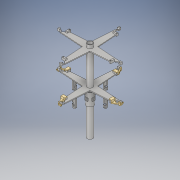
# Autodesk Inventor part: Center beam
Saved by Autodesk Inventor 2018.1 (Build 221171000, 171)
## iProperties
Created: 2017-09-02
Part Number: Center beam
Material: Generic
Document SubType Name: Modeling
Designer: ToreDenStore
Density: 1 g/cm^3
Appearance: Default
Author: ToreDenStore
Autodesk Inventor part; units mm, degrees
sketch "Sketch1" plane through (0, 0, 0) normal (0, 1, 0) x (-1, 0, 0)
  circle A0 centre (0, 0) radius 10
  circle A1 centre (0, 0) radius 8
  dimension "d0" = 20
  dimension "d1" = 2
  constraints: 2 centre point, 2 coincident
  measures "d0" diameter of A0
  measures "d1" radial gap between concentric circles of A0 A1
extrude "Extrusion1" add sketch "Sketch1" along normal blind 300
ref_plane "Work Plane1" through (0, 105, 0) normal (0, -1, 0) x (1, 0, 0)
sketch "Sketch2" plane through (0, 105, 0) normal (0, -1, 0) x (1, 0, 0)
  circle A0 centre (0, 0) radius 12.5
  circle A1 centre (0, 0) radius 10 projected
  dimension "d5" = 25
  constraints: 1 centre point, 1 coincident
  measures "d5" diameter of A0
extrude "Extrusion2" add sketch "Sketch2" against normal blind 45
ref_plane "Work Plane8" through (0, 127.5, 0) normal (0, 1, 0) x (1, 0, 0)
sketch "Sketch19" plane through (0, 127.5, 0) normal (0, 1, 0) x (1, 0, 0)
  circle A0 centre (0, 0) radius 12.5
  line L0 (-5, 11.456439) -> (-5, 14.456439)
  line L1 (-5, 14.456439) -> (5, 14.456439)
  line L2 (5, 14.456439) -> (5, 11.456439)
  line L3 (0, 19.847727) -> (0, -17.891288)
  dimension "d107" = 10
  dimension "d108" = 3
  dimension "d109" = 5
  constraints: 6 end point, 2 perpendicular, 2 point on circle, 1 vertical
  measures "d107" distance of L0.end L1.end
  measures "d108" distance of L1.end L2.end
  measures "d109" distance between parallel lines of L2 L3
extrude "Extrusion12" add sketch "Sketch19" along normal mid plane 10 contours A0 L3 L1 L2 | A0 L0 L1 L3
sketch "Sketch20" plane through (5, 132.5, -14.456439) normal (0, 0, -1) x (-1, 0, 0)
  line L0 (0, 0) -> (10, 0) projected
  line L1 (10, -10) -> (10, 0) projected
  point P0 (5, -132.5)
  point P1 (5, -6)
  dimension "d112" = 6
  dimension "d113" = 5
  measures "d112" distance from line of L0 point (5, -6)
  measures "d113" distance from line of point (5, -6) L1
hole "Hole4" at (0, 126.5, -14.456439) direction (0, 0, 1) diameter 5 depth 8 tip angle 118
pattern_circular "Circular Pattern6" count 4 over 360 about axis through (0, 0, 0) along (0, 1, 0) of "Hole4", "Extrusion12"
ref_plane "Work Plane9" through (0, 160, 0) normal (0, 1, 0) x (1, 0, 0)
sketch "Sketch3" plane through (0, 160, 0) normal (0, 1, 0) x (1, 0, 0)
  circle A0 centre (0, 0) radius 10
  line L0 (0, 0) -> (-10, 0) construction
  line L1 (-15, 0) -> (-7.98058, 100.557087)
  line L2 (7.98058, 100.557087) -> (15, 0)
  line L3 (15, 0) -> (10, 0)
  line L4 (0, 0) -> (0, 100) construction
  arc A1 (7.98058, 100.557087) -> (-7.98058, 100.557087) centre (0, 100) ccw
  circle A2 centre (0, 100) radius 5
  line L5 (10, 0) -> (0, 0) construction
  line L6 (-10, 0) -> (-15, 0)
  dimension "d9" = 15
  dimension "d10" = 100
  dimension "d11" = 8
  dimension "d12" = 10
  constraints: 14 end point, 4 collinear, 4 point on circle, 2 centre point, 2 coincident, 2 horizontal, 2 tangent, 1 equal length, 1 point on line, 1 vertical
  measures "d9" distance of L2.end L0.start
  measures "d10" distance of L0.start L4.end
  measures "d11" radius of A1
  measures "d12" diameter of A2
extrude "Extrusion3" add sketch "Sketch3" along normal blind 3 contours A0 L6 L1 A1 L2 L3
pattern_circular "Circular Pattern1" count 4 over 360 about axis through (0, 0, 0) along (0, 1, 0) of "Extrusion3"
sketch "Sketch9" plane through (0, 163, 0) normal (0, 1, 0) x (1, 0, 0)
  circle A0 centre (0, 100) radius 5
  arc A1 (7.98058, 100.557087) -> (-7.98058, 100.557087) centre (0, 100) ccw
  line L0 (0, 108) -> (0, 105)
  line L1 (0, 95) -> (0, 90)
  line L2 (0, 90) -> (8.717521, 90)
  line L3 (14.021243, 14.021243) -> (7.98058, 100.557087)
  point P0 (0, 0)
  dimension "d59" = 5
  constraints: 6 end point, 3 point on circle, 3 point on line, 1 perpendicular
  measures "d59" distance of L1.start L1.end
extrude "Extrusion7" cut sketch "Sketch9" against normal blind 5 contours A0 L0 A1 L3 L2 L1
sketch "Sketch11" plane through (0, 163, 0) normal (0, 1, 0) x (1, 0, 0)
  line L0 (0, 90) -> (8.717521, 90)
  line L1 (8.717521, 90) -> (13.717521, 90)
  line L2 (13.717521, 90) -> (13.717521, 84)
  line L3 (13.717521, 84) -> (9.136353, 84)
  arc A0 (0, 108) -> (-7.98058, 100.557087) centre (0, 100) ccw
  line L4 (0, 108) -> (0, 113)
  line L5 (0, 113) -> (-6, 113)
  line L6 (-6, 113) -> (-6, 105.291503)
  line L7 (14.021243, 14.021243) -> (8.717521, 90)
  point P0 (0, 0)
  dimension "d62" = 5
  dimension "d63" = 6
  dimension "d64" = 5
  dimension "d65" = 6
  constraints: 12 end point, 4 perpendicular, 1 horizontal, 1 point on circle, 1 point on line, 1 vertical
  measures "d62" distance of L0.end L1.end
  measures "d63" distance of L1.end L2.end
  measures "d64" distance of L4.start L4.end
  measures "d65" distance of L4.end L5.end
extrude "Extrusion8" add sketch "Sketch11" against normal blind 3
sketch "Sketch13" plane through (0, 163, 0) normal (0, 1, 0) x (1, 0, 0)
  line L0 (0, 113) -> (0, 105)
  line L1 (-6, 113) -> (0, 113)
  arc A0 (-6, 105.291503) -> (-7.98058, 100.557087) centre (0, 100) ccw
  line L2 (13.717521, 90) -> (0, 90)
  line L3 (13.717521, 90) -> (13.717521, 84)
  line L4 (13.717521, 84) -> (9.136353, 84)
  line L5 (14.021243, 14.021243) -> (9.136353, 84)
  circle A1 centre (0, 100) radius 5
  line L6 (-6, 105.291503) -> (-6, 113)
  arc A2 (-6, 105.291503) -> (-7.98058, 100.557087) centre (0, 100) ccw
  line L7 (-3, 105.291503) -> (-3, 104)
  arc A3 (0, 105) -> (0, 95) centre (0, 100) ccw
  line L8 (9.136353, 84) -> (0, 84)
  line L9 (0, 84) -> (0, 90)
  point P0 (0, 0)
  point P1 (7.98058, 100.557087)
  constraints: 6 end point, 2 vertical, 1 horizontal, 1 point on circle
sketch "Sketch13 outline for Extrusion9" plane through (0, 163, 0) normal (0, 1, 0) x (1, 0, 0)
  line L0 (0, 105) -> (0, 113)
  arc A0 (-3, 104) -> (0, 105) centre (0, 100) cw
  line L1 (-6, 105.291503) -> (-3, 104)
  line L2 (-6, 113) -> (-6, 105.291503)
  line L3 (0, 113) -> (-6, 113)
  line L4 (0, 84) -> (13.717521, 84)
  line L5 (13.717521, 84) -> (13.717521, 90)
  line L6 (13.717521, 90) -> (0, 90)
  line L7 (0, 90) -> (0, 84)
extrude "Extrusion9" add sketch "Sketch13 outline for Extrusion9" along normal blind 5
sketch "Sketch21" plane through (0, 168, 0) normal (0, 1, 0) x (1, 0, 0)
  line L0 (13.717521, 84) -> (13.717521, 90)
  line L1 (13.717521, 90) -> (0, 90)
  point P0 (0, 0)
  point P1 (10.717521, 87)
  dimension "d141" = 3
  dimension "d142" = 3
  measures "d141" distance from line of L1 point (10.718, 87)
  measures "d142" distance from line of L0 point (10.718, 87)
hole "Hole5" at (10.717521, 168, -87) direction (0, -1, 0) diameter 3 depth 4
sketch "Sketch22" plane through (10.717521, 164, -87) normal (0, 1, 0) x (1, 0, 0)
  circle A0 centre (0, 0) radius 1.5 projected
  point P0 (-10.717521, -87)
extrude "Extrusion15" add sketch "Sketch22" along normal blind 4 separate body
sketch "Sketch23" plane through (10.717521, 168, -87) normal (0, 1, 0) x (1, 0, 0)
  line L0 (3, 3) -> (-10.717521, 3)
  line L1 (3, -3) -> (3, 3)
  line L2 (-10.717521, -3) -> (3, -3)
  line L3 (-10.717521, 3) -> (-10.717521, -3)
  point P0 (-10.717521, -87)
extrude "Extrusion16" add sketch "Sketch23" along normal blind 3 bodies 2
sketch "Sketch18" plane through (0, 163, 0) normal (0, 1, 0) x (1, 0, 0)
  arc A0 (-3, 104) -> (0, 95) centre (0, 100) ccw projected
  circle A1 centre (0, 100) radius 8
  point P0 (0, 0)
  dimension "d97" = 16
  constraints: 1 centre point, 1 coincident
  measures "d97" diameter of A1
extrude "Extrusion11" cut sketch "Sketch18" along normal blind 5 bodies 1
sketch "Sketch24" plane through (13.717521, 168, -90) normal (0, 0, -1) x (-1, 0, 0)
  line L0 (13.717521, 3) -> (0, 3)
  line L1 (0, 0) -> (0, -8)
  line L2 (0, 0) -> (0, 3)
  line L3 (13.717521, 0) -> (13.717521, 3)
  line L4 (13.717521, -5) -> (13.717521, 0)
  line L5 (3.717521, -8) -> (23.717521, -8)
  line L6 (0, -8) -> (4.581168, -8)
  line L7 (13.717521, -5) -> (13.717521, -8)
  point P0 (13.717521, -168)
  constraints: 2 end point, 1 midpoint
extrude "Extrusion17" add sketch "Sketch24" along normal blind 3 bodies 2
sketch "Sketch25" plane through (0, 160, -90) normal (0, -1, 0) x (1, 0, 0)
  arc A0 (0, -5) -> (0, -15) centre (0, -10) ccw
  line L0 (0, -23) -> (0, -15)
  line L1 (0, -5) -> (0, 0)
  line L2 (13.717521, -3) -> (0, -3)
  circle A1 centre (0, -10) radius 5
  line L3 (0, -23) -> (3, -23)
  circle A2 centre (0, -10) radius 8
  line L4 (13.717521, -3) -> (6.808814, -14.200006)
  line L5 (3, -23) -> (3, -17.416198)
  point P0 (0, 90)
  dimension "d172" = 10
  dimension "d173" = 3
  dimension "d174" = 16
  constraints: 6 end point, 2 centre point, 2 coincident, 2 point on circle, 1 horizontal, 1 tangent, 1 vertical
  measures "d172" diameter of A1
  measures "d173" distance of L0.start L3.end
  measures "d174" diameter of A2
extrude "Extrusion22" add sketch "Sketch25" against normal blind 3 contours L1 L2 A2 L0 A1 | A2 L5 L3 L0 | L2 L4 A2 bodies 2
sketch "Sketch30" plane through (0, 160, -90) normal (0, -1, 0) x (1, 0, 0)
  line L0 (3, -23) -> (3, -17.416198)
  line L1 (0, -23) -> (3, -23)
  line L2 (-6, -23) -> (0, -23)
  line L3 (-6, -15.291503) -> (-6, -23)
  line L4 (3, -19) -> (-6, -19)
  point P0 (0, 90)
  dimension "d177" = 4
  constraints: 2 end point, 2 point on line, 1 perpendicular
  measures "d177" distance between parallel lines of L1 L4
extrude "Extrusion23" add sketch "Sketch30" along normal blind 3 bodies 2
sketch "Sketch31" plane through (0, 163, -90) normal (0, 1, 0) x (1, 0, 0)
  line L0 (0, 18) -> (0, 23)
  line L1 (3, 23) -> (0, 23)
  line L2 (3, 17.416198) -> (3, 23)
  line L3 (0, 18) -> (0, 15)
  line L4 (0, 18) -> (3, 17.416198)
  point P0 (0, -90)
  constraints: 2 end point
extrude "Extrusion24" add sketch "Sketch31" along normal blind 5 bodies 2
sketch "Sketch32" plane through (0, 163, -90) normal (0, 1, 0) x (1, 0, 0)
  arc A0 (0, 5) -> (0, 15) centre (0, 10) ccw projected
  circle A1 centre (0, 10) radius 8
  circle A2 centre (0, 10) radius 5
  point P0 (0, -90)
  dimension "d182" = 16
  dimension "d183" = 10
  constraints: 2 centre point, 2 coincident
  measures "d182" diameter of A1
  measures "d183" diameter of A2
extrude "Extrusion25" cut sketch "Sketch32" along normal blind 10 bodies 2
sketch "Sketch33" plane through (0, 160, -113) normal (0, 0, -1) x (-1, 0, 0)
  line L0 (-3, 0) -> (-3, 3) projected
  line L1 (-3, 3) -> (-3, 8) projected
  line L2 (-3, 4) -> (9, 4)
  line L3 (6, 3) -> (6, 8) projected
  line L4 (-3, 1) -> (9, 1)
  line L5 (10, 3) -> (-10, 3) projected
  line L6 (9, 4) -> (9, 1)
  point P0 (0, -160)
  dimension "d186" = 3
  dimension "d187" = 4
  dimension "d188" = 3
  constraints: 6 end point, 2 point on line, 1 horizontal, 1 parallel, 1 vertical
  measures "d186" distance from line of L3 L2.end
  measures "d187" distance of L1.end L2.start
  measures "d188" distance between parallel lines of L2 L4
extrude "Extrusion26" add sketch "Sketch33" along normal blind 1 bodies 2
sketch "Sketch34" plane through (-9, 164, -113) normal (0, 1, 0) x (1, 0, 0)
  line L0 (3, 0) -> (3, -7.708497)
  line L1 (0, 0) -> (9, 0)
  line L2 (0, 0) -> (3, -1)
  point P0 (9, -113)
  dimension "d191" = 1
  constraints: 2 end point, 1 point on line
  measures "d191" distance of L2.end L0.start
extrude "Extrusion27" add sketch "Sketch34" against normal blind 3 bodies 2
sketch "Sketch35" plane through (0, 160, 0) normal (0, -1, 0) x (1, 0, 0)
  arc A0 (13.717521, -87) -> (10.717521, -90) centre (10.717521, -87) ccw construction
  line L0 (0, -90) -> (13.717521, -90)
  line L1 (13.717521, -90) -> (13.717521, -84)
  arc A1 (10.717521, -90) -> (13.717521, -87) centre (10.717521, -87) ccw
  point P0 (0, 0)
  dimension "d194" = 3
  dimension "d195" = 3
  dimension "d196" = 6
  constraints: 4 point on circle, 2 centre point, 1 midpoint, 1 point on line
  measures "d194" distance from line of L0 A0.centre
  measures "d195" distance from line of L1 A0.centre
  measures "d196" diameter of A0
extrude "Extrusion28" cut sketch "Sketch35" against normal blind 8 bodies 1
pattern_circular "Circular Pattern5" count 4 over 360 about axis through (0, 0, 0) along (0, 1, 0) of "Extrusion7", "Extrusion8", "Extrusion9", "Extrusion11", "Hole5" bodies 1
pattern_circular "Circular Pattern8" count 4 over 360 about axis through (0, 0, 0) along (0, 1, 0) of "Extrusion15", "Extrusion16", "Extrusion11", "Extrusion17", "Extrusion22", "Extrusion23", "Extrusion24", "Extrusion25", "Extrusion26", "Extrusion27", "Extrusion28" bodies 2
ref_plane "Work Plane10" through (-5, 132.5, 54.456439) normal (0, 0, 1) x (1, 0, 0)
sketch "Sketch7" plane through (-5, 125, 54.456439) normal (0, 0, 1) x (1, 0, 0)
  line L0 (11, 1.5) -> (11, 35)
  arc A0 (-1, 1.5) -> (11, 1.5) centre (5, 1.5) ccw
  line L1 (-1, 1.5) -> (-1, 35)
  circle A1 centre (5, 1.5) radius 2.5 projected
  line L2 (-5, 35) -> (15, 35) projected
  point P0 (5, -125)
  dimension "d0" = 20
  dimension "d44" = 6
  dimension "d126" = 0
  constraints: 4 end point, 2 point on circle, 2 point on line, 2 tangent, 2 vertical, 1 centre point
  measures "d44" radius of A0
  measures "d126" distance of A1.centre A0.centre
extrude "Extrusion13" add sketch "Sketch7" along normal blind 5 bodies 1
sketch "Sketch8" plane through (-5, 125, 59.456439) normal (0, 0, 1) x (1, 0, 0)
  line L0 (-1, 35) -> (-1, 1.5) projected
  arc A0 (2.5, 6.5) -> (0, 9) centre (0, 6.5) ccw
  line L1 (0, 9) -> (-1, 9)
  line L2 (7.5, 1.5) -> (7.5, 6.5)
  arc A1 (7.5, 6.5) -> (0, 14) centre (0, 6.5) ccw
  line L3 (0, 14) -> (-1, 14)
  line L4 (2.5, 6.5) -> (2.5, 1.5)
  circle A2 centre (5, 1.5) radius 2.5 projected
  point P0 (5, -125)
  dimension "d129" = 5
  dimension "d130" = 1
  dimension "d131" = 5
  constraints: 8 end point, 6 point on circle, 5 parallel, 4 tangent, 2 centre point, 2 point on line, 1 perpendicular
  measures "d129" distance of L2.start L2.end
  measures "d130" distance of L1.start L1.end
  measures "d131" distance between parallel lines of L2 L4
extrude "Extrusion14" cut sketch "Sketch8" against normal blind 5 contours L3 A1 L2 A2 L4 A0 L1 L0 bodies 1
pattern_circular "Circular Pattern7" count 4 over 360 about axis through (0, 0, 0) along (0, 1, 0) of "Extrusion13", "Extrusion14" bodies 1
pattern_linear "Rectangular Pattern3" count 2 spacing 125 along (0, 1, 0) of "Extrusion7", "Extrusion8", "Extrusion9", "Extrusion11", "Circular Pattern5", "Extrusion3", "Circular Pattern1", "Hole5" bodies 1
equation "\"d142\" = d141"
body "Solid1"
body "Solid2"
